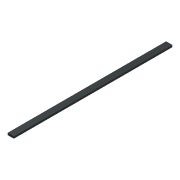
# Autodesk Inventor part: BackPlates
Saved by Autodesk Inventor 2018 (Build 220112000, 112)
## iProperties
Created: 2020-03-01
Part Number: BackPlates
Material: Iron, Cast
Document SubType Name: Modeling
Designer: Spark
Density: 7.15 g/cm^3
Appearance: Iron Gray
Author: Spark
Autodesk Inventor part; units mm, degrees
ref_plane "YZ Plane" through (0, 0, 0) normal (1, 0, 0) x (0, 1, 0)
ref_plane "XZ Plane" through (0, 0, 0) normal (0, 1, 0) x (-1, 0, 0)
ref_plane "XY Plane" through (0, 0, 0) normal (0, 0, 1) x (1, 0, 0)
sketch "Sketch1" plane through (0, 0, 0) normal (0, 0, 1) x (1, 0, 0)
  line L0 (0, 0) -> (30, 0)
  line L1 (30, 0) -> (30, 798.434)
  line L2 (30, 798.434) -> (0, 798.434)
  line L3 (0, 798.434) -> (0, 0)
  dimension "d0" = 30
  dimension "d1" = 798.434
  constraints: 8 end point, 2 parallel, 1 horizontal, 1 perpendicular
  measures "d0" distance of L2.end L1.end
  measures "d1" distance of L1.end L0.end
extrude "Extrusion1" add sketch "Sketch1" along normal blind 10
sketch "Sketch5" plane through (0, 0, 0) normal (0, 0, -1) x (-1, 0, 0)
  line L0 (0, 0) -> (-30, 0) projected
  line L1 (-30, 798.434) -> (0, 798.434) projected
  line L2 (-30, 0) -> (-30, 798.434) projected
  point P0 (-15, 50)
  point P1 (-15, 698.434)
  dimension "d25" = 50
  dimension "d26" = 100
  dimension "d27" = 15
  dimension "d28" = 15
  measures "d25" distance from line of L0 point (-15, 50)
  measures "d26" distance from line of point (-15, 698.434) L1
  measures "d27" distance from line of L2 point (-15, 698.434)
  measures "d28" distance from line of L2 point (-15, 50)
hole "Hole2" at (15, 50, 0) at (15, 698.434, 0) direction (0, 0, 1) diameter 3 end through all countersink diameter 6.1 countersink angle 90
body "Solid1"
